Autodesk Inventor part; units mm, degrees
(part 2 of 2)
sketch "Sketch6" plane through (0, 0, 3) normal (0, 0, 1) x (1, 0, 0)
  circle A0 centre (23.8475, 52.0575) radius 1.738 projected
  circle A1 centre (25.1175, 3.7975) radius 1.738 projected
  circle A2 centre (-26.9525, 36.8175) radius 1.738 projected
  line L0 (23.8475, 52.0575) -> (25.1175, 3.7975) construction
  line L1 (20.0988, 51.9588) -> (21.3688, 3.6988)
  line L2 (28.8662, 3.8962) -> (27.5962, 52.1562)
  arc A3 (27.5962, 52.1562) -> (20.0988, 51.9588) centre (23.8475, 52.0575) ccw
  arc A4 (21.3688, 3.6988) -> (28.8662, 3.8962) centre (25.1175, 3.7975) ccw
  line L3 (23.8475, 52.0575) -> (-26.9525, 36.8175) construction
  line L4 (22.7699, 55.6493) -> (-28.0301, 40.4093)
  line L5 (-25.8749, 33.2257) -> (24.9251, 48.4657)
  arc A5 (24.9251, 48.4657) -> (22.7699, 55.6493) centre (23.8475, 52.0575) ccw
  arc A6 (-28.0301, 40.4093) -> (-25.8749, 33.2257) centre (-26.9525, 36.8175) ccw
  line L6 (-26.9525, 36.8175) -> (25.1175, 3.7975) construction
  line L7 (-24.9442, 39.9844) -> (27.1258, 6.9644)
  line L8 (23.1092, 0.6306) -> (-28.9608, 33.6506)
  arc A7 (-24.9442, 39.9844) -> (-28.9608, 33.6506) centre (-26.9525, 36.8175) ccw
  arc A8 (23.1092, 0.6306) -> (27.1258, 6.9644) centre (25.1175, 3.7975) ccw
  line L9 (27.1, 62.12) -> (27.1, 54.72) projected
  line L10 (-27.1, -6.2) -> (27.1, -6.2)
  line L11 (27.1, -6.2) -> (27.1, 62.12)
  line L12 (27.1, 62.12) -> (-27.1, 62.12)
  line L13 (-27.1, 62.12) -> (-27.1, -6.2)
  line L14 (27.1, 62.12) -> (-27.1, 62.12) projected
  line L15 (-27.1, 62.12) -> (-27.1, 54.72) projected
  line L16 (-27.1, 54.72) -> (27.1, 54.72) projected
  line L17 (27.1, 54.72) -> (27.1, 62.12) projected
  line L18 (-0.72, 56.35) -> (-2.32, 56.35) projected
  line L19 (-2.32, 56.35) -> (-2.32, 57.95) projected
  line L20 (-2.32, 57.95) -> (-0.72, 57.95) projected
  line L21 (-0.72, 57.95) -> (-0.72, 56.35) projected
  line L22 (-0.72, 58.89) -> (-2.32, 58.89) projected
  line L23 (-2.32, 58.89) -> (-2.32, 60.49) projected
  line L24 (-2.32, 60.49) -> (-0.72, 60.49) projected
  line L25 (-0.72, 60.49) -> (-0.72, 58.89) projected
  line L26 (-3.26, 56.35) -> (-4.86, 56.35) projected
  line L27 (-4.86, 56.35) -> (-4.86, 57.95) projected
  line L28 (-4.86, 57.95) -> (-3.26, 57.95) projected
  line L29 (-3.26, 57.95) -> (-3.26, 56.35) projected
  line L30 (-3.26, 58.89) -> (-4.86, 58.89) projected
  line L31 (-4.86, 58.89) -> (-4.86, 60.49) projected
  line L32 (-4.86, 60.49) -> (-3.26, 60.49) projected
  line L33 (-3.26, 60.49) -> (-3.26, 58.89) projected
  line L34 (-5.8, 56.35) -> (-7.4, 56.35) projected
  line L35 (-7.4, 56.35) -> (-7.4, 57.95) projected
  line L36 (-7.4, 57.95) -> (-5.8, 57.95) projected
  line L37 (-5.8, 57.95) -> (-5.8, 56.35) projected
  line L38 (-5.8, 58.89) -> (-7.4, 58.89) projected
  line L39 (-7.4, 58.89) -> (-7.4, 60.49) projected
  line L40 (-7.4, 60.49) -> (-5.8, 60.49) projected
  line L41 (-5.8, 60.49) -> (-5.8, 58.89) projected
  line L42 (-8.34, 56.35) -> (-9.94, 56.35) projected
  line L43 (-9.94, 56.35) -> (-9.94, 57.95) projected
  line L44 (-9.94, 57.95) -> (-8.34, 57.95) projected
  line L45 (-8.34, 57.95) -> (-8.34, 56.35) projected
  line L46 (-8.34, 58.89) -> (-9.94, 58.89) projected
  line L47 (-9.94, 58.89) -> (-9.94, 60.49) projected
  line L48 (-9.94, 60.49) -> (-8.34, 60.49) projected
  line L49 (-8.34, 60.49) -> (-8.34, 58.89) projected
  line L50 (-10.88, 56.35) -> (-12.48, 56.35) projected
  line L51 (-12.48, 56.35) -> (-12.48, 57.95) projected
  line L52 (-12.48, 57.95) -> (-10.88, 57.95) projected
  line L53 (-10.88, 57.95) -> (-10.88, 56.35) projected
  line L54 (-10.88, 58.89) -> (-12.48, 58.89) projected
  line L55 (-12.48, 58.89) -> (-12.48, 60.49) projected
  line L56 (-12.48, 60.49) -> (-10.88, 60.49) projected
  line L57 (-10.88, 60.49) -> (-10.88, 58.89) projected
  line L58 (-13.42, 56.35) -> (-15.02, 56.35) projected
  line L59 (-15.02, 56.35) -> (-15.02, 57.95) projected
  line L60 (-15.02, 57.95) -> (-13.42, 57.95) projected
  line L61 (-13.42, 57.95) -> (-13.42, 56.35) projected
  line L62 (-13.42, 58.89) -> (-15.02, 58.89) projected
  line L63 (-15.02, 58.89) -> (-15.02, 60.49) projected
  line L64 (-15.02, 60.49) -> (-13.42, 60.49) projected
  line L65 (-13.42, 60.49) -> (-13.42, 58.89) projected
  line L66 (-15.96, 56.35) -> (-17.56, 56.35) projected
  line L67 (-17.56, 56.35) -> (-17.56, 57.95) projected
  line L68 (-17.56, 57.95) -> (-15.96, 57.95) projected
  line L69 (-15.96, 57.95) -> (-15.96, 56.35) projected
  line L70 (-15.96, 58.89) -> (-17.56, 58.89) projected
  line L71 (-17.56, 58.89) -> (-17.56, 60.49) projected
  line L72 (-17.56, 60.49) -> (-15.96, 60.49) projected
  line L73 (-15.96, 60.49) -> (-15.96, 58.89) projected
  line L74 (-18.5, 56.35) -> (-20.1, 56.35) projected
  line L75 (-20.1, 56.35) -> (-20.1, 57.95) projected
  line L76 (-20.1, 57.95) -> (-18.5, 57.95) projected
  line L77 (-18.5, 57.95) -> (-18.5, 56.35) projected
  line L78 (-18.5, 58.89) -> (-20.1, 58.89) projected
  line L79 (-20.1, 58.89) -> (-20.1, 60.49) projected
  line L80 (-20.1, 60.49) -> (-18.5, 60.49) projected
  line L81 (-18.5, 60.49) -> (-18.5, 58.89) projected
  line L82 (-21.04, 56.35) -> (-22.64, 56.35) projected
  line L83 (-22.64, 56.35) -> (-22.64, 57.95) projected
  line L84 (-22.64, 57.95) -> (-21.04, 57.95) projected
  line L85 (-21.04, 57.95) -> (-21.04, 56.35) projected
  line L86 (-21.04, 58.89) -> (-22.64, 58.89) projected
  line L87 (-22.64, 58.89) -> (-22.64, 60.49) projected
  line L88 (-22.64, 60.49) -> (-21.04, 60.49) projected
  line L89 (-21.04, 60.49) -> (-21.04, 58.89) projected
  line L90 (-23.58, 56.35) -> (-25.18, 56.35) projected
  line L91 (-25.18, 56.35) -> (-25.18, 57.95) projected
  line L92 (-25.18, 57.95) -> (-23.58, 57.95) projected
  line L93 (-23.58, 57.95) -> (-23.58, 56.35) projected
  line L94 (-23.58, 58.89) -> (-25.18, 58.89) projected
  line L95 (-25.18, 58.89) -> (-25.18, 60.49) projected
  line L96 (-25.18, 60.49) -> (-23.58, 60.49) projected
  line L97 (-23.58, 60.49) -> (-23.58, 58.89) projected
  line L98 (25.18, 56.35) -> (23.58, 56.35) projected
  line L99 (23.58, 56.35) -> (23.58, 57.95) projected
  line L100 (23.58, 57.95) -> (25.18, 57.95) projected
  line L101 (25.18, 57.95) -> (25.18, 56.35) projected
  line L102 (25.18, 58.89) -> (23.58, 58.89) projected
  line L103 (23.58, 58.89) -> (23.58, 60.49) projected
  line L104 (23.58, 60.49) -> (25.18, 60.49) projected
  line L105 (25.18, 60.49) -> (25.18, 58.89) projected
  line L106 (22.64, 56.35) -> (21.04, 56.35) projected
  line L107 (21.04, 56.35) -> (21.04, 57.95) projected
  line L108 (21.04, 57.95) -> (22.64, 57.95) projected
  line L109 (22.64, 57.95) -> (22.64, 56.35) projected
  line L110 (22.64, 58.89) -> (21.04, 58.89) projected
  line L111 (21.04, 58.89) -> (21.04, 60.49) projected
  line L112 (21.04, 60.49) -> (22.64, 60.49) projected
  line L113 (22.64, 60.49) -> (22.64, 58.89) projected
  line L114 (20.1, 56.35) -> (18.5, 56.35) projected
  line L115 (18.5, 56.35) -> (18.5, 57.95) projected
  line L116 (18.5, 57.95) -> (20.1, 57.95) projected
  line L117 (20.1, 57.95) -> (20.1, 56.35) projected
  line L118 (20.1, 58.89) -> (18.5, 58.89) projected
  line L119 (18.5, 58.89) -> (18.5, 60.49) projected
  line L120 (18.5, 60.49) -> (20.1, 60.49) projected
  line L121 (20.1, 60.49) -> (20.1, 58.89) projected
  line L122 (17.56, 56.35) -> (15.96, 56.35) projected
  line L123 (15.96, 56.35) -> (15.96, 57.95) projected
  line L124 (15.96, 57.95) -> (17.56, 57.95) projected
  line L125 (17.56, 57.95) -> (17.56, 56.35) projected
  line L126 (17.56, 58.89) -> (15.96, 58.89) projected
  line L127 (15.96, 58.89) -> (15.96, 60.49) projected
  line L128 (15.96, 60.49) -> (17.56, 60.49) projected
  line L129 (17.56, 60.49) -> (17.56, 58.89) projected
  line L130 (15.02, 56.35) -> (13.42, 56.35) projected
  line L131 (13.42, 56.35) -> (13.42, 57.95) projected
  line L132 (13.42, 57.95) -> (15.02, 57.95) projected
  line L133 (15.02, 57.95) -> (15.02, 56.35) projected
  line L134 (15.02, 58.89) -> (13.42, 58.89) projected
  line L135 (13.42, 58.89) -> (13.42, 60.49) projected
  line L136 (13.42, 60.49) -> (15.02, 60.49) projected
  line L137 (15.02, 60.49) -> (15.02, 58.89) projected
  line L138 (12.48, 56.35) -> (10.88, 56.35) projected
  line L139 (10.88, 56.35) -> (10.88, 57.95) projected
  line L140 (10.88, 57.95) -> (12.48, 57.95) projected
  line L141 (12.48, 57.95) -> (12.48, 56.35) projected
  line L142 (12.48, 58.89) -> (10.88, 58.89) projected
  line L143 (10.88, 58.89) -> (10.88, 60.49) projected
  line L144 (10.88, 60.49) -> (12.48, 60.49) projected
  line L145 (12.48, 60.49) -> (12.48, 58.89) projected
  line L146 (9.94, 56.35) -> (8.34, 56.35) projected
  line L147 (8.34, 56.35) -> (8.34, 57.95) projected
  line L148 (8.34, 57.95) -> (9.94, 57.95) projected
  line L149 (9.94, 57.95) -> (9.94, 56.35) projected
  line L150 (9.94, 58.89) -> (8.34, 58.89) projected
  line L151 (8.34, 58.89) -> (8.34, 60.49) projected
  line L152 (8.34, 60.49) -> (9.94, 60.49) projected
  line L153 (9.94, 60.49) -> (9.94, 58.89) projected
  line L154 (7.4, 56.35) -> (5.8, 56.35) projected
  line L155 (5.8, 56.35) -> (5.8, 57.95) projected
  line L156 (5.8, 57.95) -> (7.4, 57.95) projected
  line L157 (7.4, 57.95) -> (7.4, 56.35) projected
  line L158 (7.4, 58.89) -> (5.8, 58.89) projected
  line L159 (5.8, 58.89) -> (5.8, 60.49) projected
  line L160 (5.8, 60.49) -> (7.4, 60.49) projected
  line L161 (7.4, 60.49) -> (7.4, 58.89) projected
  line L162 (4.86, 56.35) -> (3.26, 56.35) projected
  line L163 (3.26, 56.35) -> (3.26, 57.95) projected
  line L164 (3.26, 57.95) -> (4.86, 57.95) projected
  line L165 (4.86, 57.95) -> (4.86, 56.35) projected
  line L166 (4.86, 58.89) -> (3.26, 58.89) projected
  line L167 (3.26, 58.89) -> (3.26, 60.49) projected
  line L168 (3.26, 60.49) -> (4.86, 60.49) projected
  line L169 (4.86, 60.49) -> (4.86, 58.89) projected
  line L170 (2.32, 56.35) -> (0.72, 56.35) projected
  line L171 (0.72, 56.35) -> (0.72, 57.95) projected
  line L172 (0.72, 57.95) -> (2.32, 57.95) projected
  line L173 (2.32, 57.95) -> (2.32, 56.35) projected
  line L174 (2.32, 58.89) -> (0.72, 58.89) projected
  line L175 (0.72, 58.89) -> (0.72, 60.49) projected
  line L176 (0.72, 60.49) -> (2.32, 60.49) projected
  line L177 (2.32, 60.49) -> (2.32, 58.89) projected
  line L178 (-27.1, 1.2) -> (-27.1, -6.2) projected
  line L179 (-27.1, -6.2) -> (27.1, -6.2) projected
  line L180 (27.1, -6.2) -> (27.1, 1.2) projected
  line L181 (27.1, 1.2) -> (-27.1, 1.2) projected
  line L182 (2.32, -2.03) -> (0.72, -2.03) projected
  line L183 (0.72, -2.03) -> (0.72, -0.43) projected
  line L184 (0.72, -0.43) -> (2.32, -0.43) projected
  line L185 (2.32, -0.43) -> (2.32, -2.03) projected
  line L186 (2.32, -4.57) -> (0.72, -4.57) projected
  line L187 (0.72, -4.57) -> (0.72, -2.97) projected
  line L188 (0.72, -2.97) -> (2.32, -2.97) projected
  line L189 (2.32, -2.97) -> (2.32, -4.57) projected
  line L190 (4.86, -2.03) -> (3.26, -2.03) projected
  line L191 (3.26, -2.03) -> (3.26, -0.43) projected
  line L192 (3.26, -0.43) -> (4.86, -0.43) projected
  line L193 (4.86, -0.43) -> (4.86, -2.03) projected
  line L194 (4.86, -4.57) -> (3.26, -4.57) projected
  line L195 (3.26, -4.57) -> (3.26, -2.97) projected
  line L196 (3.26, -2.97) -> (4.86, -2.97) projected
  line L197 (4.86, -2.97) -> (4.86, -4.57) projected
  line L198 (7.4, -2.03) -> (5.8, -2.03) projected
  line L199 (5.8, -2.03) -> (5.8, -0.43) projected
  line L200 (5.8, -0.43) -> (7.4, -0.43) projected
  line L201 (7.4, -0.43) -> (7.4, -2.03) projected
  line L202 (7.4, -4.57) -> (5.8, -4.57) projected
  line L203 (5.8, -4.57) -> (5.8, -2.97) projected
  line L204 (5.8, -2.97) -> (7.4, -2.97) projected
  line L205 (7.4, -2.97) -> (7.4, -4.57) projected
  line L206 (9.94, -2.03) -> (8.34, -2.03) projected
  line L207 (8.34, -2.03) -> (8.34, -0.43) projected
  line L208 (8.34, -0.43) -> (9.94, -0.43) projected
  line L209 (9.94, -0.43) -> (9.94, -2.03) projected
  line L210 (9.94, -4.57) -> (8.34, -4.57) projected
  line L211 (8.34, -4.57) -> (8.34, -2.97) projected
  line L212 (8.34, -2.97) -> (9.94, -2.97) projected
  line L213 (9.94, -2.97) -> (9.94, -4.57) projected
  line L214 (12.48, -2.03) -> (10.88, -2.03) projected
  line L215 (10.88, -2.03) -> (10.88, -0.43) projected
  line L216 (10.88, -0.43) -> (12.48, -0.43) projected
  line L217 (12.48, -0.43) -> (12.48, -2.03) projected
  line L218 (12.48, -4.57) -> (10.88, -4.57) projected
  line L219 (10.88, -4.57) -> (10.88, -2.97) projected
  line L220 (10.88, -2.97) -> (12.48, -2.97) projected
  line L221 (12.48, -2.97) -> (12.48, -4.57) projected
  line L222 (15.02, -2.03) -> (13.42, -2.03) projected
  line L223 (13.42, -2.03) -> (13.42, -0.43) projected
  line L224 (13.42, -0.43) -> (15.02, -0.43) projected
  line L225 (15.02, -0.43) -> (15.02, -2.03) projected
  line L226 (15.02, -4.57) -> (13.42, -4.57) projected
  line L227 (13.42, -4.57) -> (13.42, -2.97) projected
  line L228 (13.42, -2.97) -> (15.02, -2.97) projected
  line L229 (15.02, -2.97) -> (15.02, -4.57) projected
  line L230 (17.56, -2.03) -> (15.96, -2.03) projected
  line L231 (15.96, -2.03) -> (15.96, -0.43) projected
  line L232 (15.96, -0.43) -> (17.56, -0.43) projected
  line L233 (17.56, -0.43) -> (17.56, -2.03) projected
  line L234 (17.56, -4.57) -> (15.96, -4.57) projected
  line L235 (15.96, -4.57) -> (15.96, -2.97) projected
  line L236 (15.96, -2.97) -> (17.56, -2.97) projected
  line L237 (17.56, -2.97) -> (17.56, -4.57) projected
  line L238 (20.1, -2.03) -> (18.5, -2.03) projected
  line L239 (18.5, -2.03) -> (18.5, -0.43) projected
  line L240 (18.5, -0.43) -> (20.1, -0.43) projected
  line L241 (20.1, -0.43) -> (20.1, -2.03) projected
  line L242 (20.1, -4.57) -> (18.5, -4.57) projected
  line L243 (18.5, -4.57) -> (18.5, -2.97) projected
  line L244 (18.5, -2.97) -> (20.1, -2.97) projected
  line L245 (20.1, -2.97) -> (20.1, -4.57) projected
  line L246 (22.64, -2.03) -> (21.04, -2.03) projected
  line L247 (21.04, -2.03) -> (21.04, -0.43) projected
  line L248 (21.04, -0.43) -> (22.64, -0.43) projected
  line L249 (22.64, -0.43) -> (22.64, -2.03) projected
  line L250 (22.64, -4.57) -> (21.04, -4.57) projected
  line L251 (21.04, -4.57) -> (21.04, -2.97) projected
  line L252 (21.04, -2.97) -> (22.64, -2.97) projected
  line L253 (22.64, -2.97) -> (22.64, -4.57) projected
  line L254 (25.18, -2.03) -> (23.58, -2.03) projected
  line L255 (23.58, -2.03) -> (23.58, -0.43) projected
  line L256 (23.58, -0.43) -> (25.18, -0.43) projected
  line L257 (25.18, -0.43) -> (25.18, -2.03) projected
  line L258 (25.18, -4.57) -> (23.58, -4.57) projected
  line L259 (23.58, -4.57) -> (23.58, -2.97) projected
  line L260 (23.58, -2.97) -> (25.18, -2.97) projected
  line L261 (25.18, -2.97) -> (25.18, -4.57) projected
  line L262 (-23.58, -2.03) -> (-25.18, -2.03) projected
  line L263 (-25.18, -2.03) -> (-25.18, -0.43) projected
  line L264 (-25.18, -0.43) -> (-23.58, -0.43) projected
  line L265 (-23.58, -0.43) -> (-23.58, -2.03) projected
  line L266 (-23.58, -4.57) -> (-25.18, -4.57) projected
  line L267 (-25.18, -4.57) -> (-25.18, -2.97) projected
  line L268 (-25.18, -2.97) -> (-23.58, -2.97) projected
  line L269 (-23.58, -2.97) -> (-23.58, -4.57) projected
  line L270 (-21.04, -2.03) -> (-22.64, -2.03) projected
  line L271 (-22.64, -2.03) -> (-22.64, -0.43) projected
  line L272 (-22.64, -0.43) -> (-21.04, -0.43) projected
  line L273 (-21.04, -0.43) -> (-21.04, -2.03) projected
  line L274 (-21.04, -4.57) -> (-22.64, -4.57) projected
  line L275 (-22.64, -4.57) -> (-22.64, -2.97) projected
  line L276 (-22.64, -2.97) -> (-21.04, -2.97) projected
  line L277 (-21.04, -2.97) -> (-21.04, -4.57) projected
  line L278 (-18.5, -2.03) -> (-20.1, -2.03) projected
  line L279 (-20.1, -2.03) -> (-20.1, -0.43) projected
  line L280 (-20.1, -0.43) -> (-18.5, -0.43) projected
  line L281 (-18.5, -0.43) -> (-18.5, -2.03) projected
  line L282 (-18.5, -4.57) -> (-20.1, -4.57) projected
  line L283 (-20.1, -4.57) -> (-20.1, -2.97) projected
  line L284 (-20.1, -2.97) -> (-18.5, -2.97) projected
  line L285 (-18.5, -2.97) -> (-18.5, -4.57) projected
  line L286 (-15.96, -2.03) -> (-17.56, -2.03) projected
  line L287 (-17.56, -2.03) -> (-17.56, -0.43) projected
  line L288 (-17.56, -0.43) -> (-15.96, -0.43) projected
  line L289 (-15.96, -0.43) -> (-15.96, -2.03) projected
  line L290 (-15.96, -4.57) -> (-17.56, -4.57) projected
  line L291 (-17.56, -4.57) -> (-17.56, -2.97) projected
  line L292 (-17.56, -2.97) -> (-15.96, -2.97) projected
  line L293 (-15.96, -2.97) -> (-15.96, -4.57) projected
  line L294 (-13.42, -2.03) -> (-15.02, -2.03) projected
  line L295 (-15.02, -2.03) -> (-15.02, -0.43) projected
  line L296 (-15.02, -0.43) -> (-13.42, -0.43) projected
  line L297 (-13.42, -0.43) -> (-13.42, -2.03) projected
  line L298 (-13.42, -4.57) -> (-15.02, -4.57) projected
  line L299 (-15.02, -4.57) -> (-15.02, -2.97) projected
  line L300 (-15.02, -2.97) -> (-13.42, -2.97) projected
  line L301 (-13.42, -2.97) -> (-13.42, -4.57) projected
  line L302 (-10.88, -2.03) -> (-12.48, -2.03) projected
  line L303 (-12.48, -2.03) -> (-12.48, -0.43) projected
  line L304 (-12.48, -0.43) -> (-10.88, -0.43) projected
  line L305 (-10.88, -0.43) -> (-10.88, -2.03) projected
  line L306 (-10.88, -4.57) -> (-12.48, -4.57) projected
  line L307 (-12.48, -4.57) -> (-12.48, -2.97) projected
  line L308 (-12.48, -2.97) -> (-10.88, -2.97) projected
  line L309 (-10.88, -2.97) -> (-10.88, -4.57) projected
  line L310 (-8.34, -2.03) -> (-9.94, -2.03) projected
  line L311 (-9.94, -2.03) -> (-9.94, -0.43) projected
  line L312 (-9.94, -0.43) -> (-8.34, -0.43) projected
  line L313 (-8.34, -0.43) -> (-8.34, -2.03) projected
  line L314 (-8.34, -4.57) -> (-9.94, -4.57) projected
  line L315 (-9.94, -4.57) -> (-9.94, -2.97) projected
  line L316 (-9.94, -2.97) -> (-8.34, -2.97) projected
  line L317 (-8.34, -2.97) -> (-8.34, -4.57) projected
  line L318 (-5.8, -2.03) -> (-7.4, -2.03) projected
  line L319 (-7.4, -2.03) -> (-7.4, -0.43) projected
  line L320 (-7.4, -0.43) -> (-5.8, -0.43) projected
  line L321 (-5.8, -0.43) -> (-5.8, -2.03) projected
  line L322 (-5.8, -4.57) -> (-7.4, -4.57) projected
  line L323 (-7.4, -4.57) -> (-7.4, -2.97) projected
  line L324 (-7.4, -2.97) -> (-5.8, -2.97) projected
  line L325 (-5.8, -2.97) -> (-5.8, -4.57) projected
  line L326 (-3.26, -2.03) -> (-4.86, -2.03) projected
  line L327 (-4.86, -2.03) -> (-4.86, -0.43) projected
  line L328 (-4.86, -0.43) -> (-3.26, -0.43) projected
  line L329 (-3.26, -0.43) -> (-3.26, -2.03) projected
  line L330 (-3.26, -4.57) -> (-4.86, -4.57) projected
  line L331 (-4.86, -4.57) -> (-4.86, -2.97) projected
  line L332 (-4.86, -2.97) -> (-3.26, -2.97) projected
  line L333 (-3.26, -2.97) -> (-3.26, -4.57) projected
  line L334 (-0.72, -2.03) -> (-2.32, -2.03) projected
  line L335 (-2.32, -2.03) -> (-2.32, -0.43) projected
  line L336 (-2.32, -0.43) -> (-0.72, -0.43) projected
  line L337 (-0.72, -0.43) -> (-0.72, -2.03) projected
  line L338 (-0.72, -4.57) -> (-2.32, -4.57) projected
  line L339 (-2.32, -4.57) -> (-2.32, -2.97) projected
  line L340 (-2.32, -2.97) -> (-0.72, -2.97) projected
  line L341 (-0.72, -2.97) -> (-0.72, -4.57) projected
  point P0 (0, 0)
  point P1 (24.4825, 27.9275)
  point P2 (-1.5525, 44.4375)
  point P3 (-0.9175, 20.3075)
  point P4 (-18.0079, 35.5858)
  point P5 (20.2278, 47.0565)
  point P6 (21.1837, 10.7326)
  point P7 (-27.1, 40.5646)
  point P8 (-28.0301, 40.4093)
  point P9 (-27.1, 33.0704)
  point P10 (27.1, 1.2)
  point P11 (27.1, 0.6144)
  point P12 (27.1, 53.924)
  dimension "d14" = 7.5
  dimension "d15" = 7.5
  dimension "d16" = 7.5
  constraints: 32 end point, 12 point on circle, 12 tangent, 6 centre point, 5 parallel, 3 midpoint, 1 horizontal, 1 perpendicular
  measures "d14" distance between parallel lines of L2 L1
  measures "d15" distance between parallel lines of L4 L5
  measures "d16" distance between parallel lines of L8 L7
extrude "Extrusion6" add sketch "Sketch6" against normal blind 3 contours A2 L13 A7 L7 L5 A6 | A2 L13 A6 A7 | L13 L4 L16 A3 L1 L5 L7 A7 | A6 L5 L7 L1 A4 L181 L8 L13 | L13 L16 L4 | L8 L181 L13 | L5 A5 L11 L7 L1 | L1 A3 L16 L11 A5 L5 | L7 L11 L181 A4 L1 | L11 A5 L2 A8 L7 | L7 A8 A4 L11 | L16 L11 A3 | L11 A3 A5
fillet "Fillet1" radius 27 4 edges at (27.1, 0.6144, 1.5) (27.1, 53.924, 1.5) (-27.1, 40.5646, 1.5) (-27.1, 33.0704, 1.5)
sketch "Sketch7" plane through (0, 0, 3) normal (0, 0, 1) x (1, 0, 0)
  circle A0 centre (23.8475, 52.0575) radius 1.738 projected
  circle A1 centre (25.1175, 3.7975) radius 1.738 projected
  circle A2 centre (-26.9525, 36.8175) radius 1.738 projected
  circle A3 centre (-26.9525, 36.8175) radius 3.5
  circle A4 centre (23.8475, 52.0575) radius 3.5
  circle A5 centre (25.1175, 3.7975) radius 3.5
  point P0 (0, 0)
  dimension "d20" = 7
  dimension "d21" = 7
  dimension "d22" = 7
  constraints: 3 centre point, 3 coincident
  measures "d20" diameter of A3
  measures "d21" diameter of A4
  measures "d22" diameter of A5
ref_plane "Work Plane2" through (-29.3543, -6.9749, -8.9) normal (0, 0, 1) x (1, 0, 0)
extrude "Extrusion7" add sketch "Sketch7" against normal up to surface (11.9 mm away)
sketch "Sketch8" plane through (0, 0, 3) normal (0, 0, 1) x (1, 0, 0)
  circle A0 centre (0, 45.04) radius 1.75
  circle A1 centre (0, 10.88) radius 1.75
  circle A2 centre (-19.4591, 10.88) radius 1.75
  circle A3 centre (-19.4591, 45.04) radius 1.75
  line L0 (27.1, 62.12) -> (-27.1, 62.12) construction
  line L1 (0, 62.12) -> (0, -6.2) construction
  line L2 (-27.1, -6.2) -> (27.1, -6.2) construction
  line L3 (0, 27.96) -> (5.3189, 27.96) construction
  line L4 (5.3189, 27.96) -> (-6.1243, 27.96) construction
  line L5 (0, 27.96) -> (0, 62.12) construction
  line L6 (0, 27.96) -> (0, -6.2) construction
  line L7 (0, 45.04) -> (-24.0346, 45.04) construction
  line L8 (0, 10.88) -> (-24.0346, 10.88) construction
  line L9 (-27.1, 1.2) -> (-27.1, 22.3753) construction
  point P0 (0, 0)
  dimension "d25" = 3.5
  dimension "d26" = 3.5
  dimension "d27" = 3.5
  dimension "d28" = 3.5
  constraints: 14 end point, 5 midpoint, 4 centre point, 3 point on line, 2 collinear, 2 horizontal, 1 perpendicular, 1 vertical
  measures "d25" diameter of A0
  measures "d26" diameter of A1
  measures "d27" diameter of A2
  measures "d28" diameter of A3
extrude "Extrusion8" cut sketch "Sketch8" against normal up to surface (3 mm away)
sketch "Sketch9" plane through (-27.1, -6.2, -7) normal (0, -1, 0) x (1, 0, 0)
  line L0 (54.2, 0) -> (54.2, 7) construction
  line L1 (55.7518, 10) -> (54.2, 10) construction
  line L2 (54.2, 0) -> (54.2, 10) construction
  line L3 (54.2, 5) -> (-8.9852, 5) construction
  line L4 (1.8855, -1.9) -> (1.8855, 10) construction
  circle A0 centre (44.2, 5) radius 1.6
  circle A1 centre (10, 5) radius 1.6
  line L5 (0, 0) -> (0, 10) projected
  point P0 (27.1, 7)
  dimension "d31" = 3.2
  dimension "d32" = 10
  dimension "d33" = 3.2
  dimension "d34" = 10
  constraints: 4 end point, 2 centre point, 2 perpendicular, 2 point on line, 1 midpoint
  measures "d31" diameter of A0
  measures "d32" distance from line of L0 A0.centre
  measures "d33" diameter of A1
  measures "d34" distance from line of L5 A1.centre
extrude "Extrusion9" cut sketch "Sketch9" against normal through all
thread "Thread1" size "M3.5x0.6" class "6H" standard "ANSI Metric M Profile" full length
thread "Thread2" size "M3.5x0.6" class "6H" standard "ANSI Metric M Profile" full length
thread "Thread3" size "M3.5x0.6" class "6H" standard "ANSI Metric M Profile" full length
thread "Thread4" size "M3.5x0.6" class "6H" standard "ANSI Metric M Profile" full length
thread "Thread5" size "M3.5x0.6" class "6H" standard "ANSI Metric M Profile" full length
thread "Thread6" size "M3.5x0.6" class "6H" standard "ANSI Metric M Profile" full length
thread "Thread7" size "M3.5x0.6" class "6H" standard "ANSI Metric M Profile" full length
thread "Thread8" size "M3.5x0.6" class "6H" standard "ANSI Metric M Profile" full length
body "Solid3"
